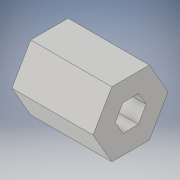
# Autodesk Inventor part: 5mm-.5in hex converter
Saved by Autodesk Inventor 2019 (Build 230136000, 136)
## iProperties
Created: 2020-09-24
Part Number: 5mm-.5in hex converter
Material: Generic
Document SubType Name: Modeling
Designer: User
Density: 1 g/cm^3
Appearance: Default
Author: User
Autodesk Inventor part; units mm, degrees
ref_plane "YZ Plane" through (0, 0, 0) normal (1, 0, 0) x (0, 1, 0)
ref_plane "XZ Plane" through (0, 0, 0) normal (0, 1, 0) x (-1, 0, 0)
ref_plane "XY Plane" through (0, 0, 0) normal (0, 0, 1) x (1, 0, 0)
sketch "Sketch1" plane through (0, 0, 0) normal (1, 0, 0) x (0, 1, 0)
  line L0 (6.35, -3.6662) -> (0, -7.3323)
  line L1 (0, -7.3323) -> (-6.35, -3.6662)
  line L2 (-6.35, -3.6662) -> (-6.35, 3.6662)
  line L3 (-6.35, 3.6662) -> (0, 7.3323)
  line L4 (0, 7.3323) -> (6.35, 3.6662)
  line L5 (6.35, 3.6662) -> (6.35, -3.6662)
  point P0 (0, 0)
  point P1 (0, 0)
  dimension "d0" = 6.35
  constraints: 12 end point, 1 coincident, 13 other
  measures "d0" distance from line of point (0, 0) L5
extrude "Extrusion1" add sketch "Sketch1" along normal blind 3.175
sketch "Sketch3" plane through (0, 0, 0) normal (-1, 0, 0) x (0, 0, 1)
  line L0 (-3.0207, 0.0407) -> (-1.475, 2.6363)
  line L1 (-1.475, 2.6363) -> (1.5456, 2.5956)
  line L2 (1.5456, 2.5956) -> (3.0207, -0.0407)
  line L3 (3.0207, -0.0407) -> (1.475, -2.6363)
  line L4 (1.475, -2.6363) -> (-1.5456, -2.5956)
  line L5 (-1.5456, -2.5956) -> (-3.0207, 0.0407)
  line L6 (-3.6662, 6.35) -> (-7.3323, 0) projected
  line L7 (-7.3323, 0) -> (-3.6662, -6.35) projected
  line L8 (-3.6662, -6.35) -> (3.6662, -6.35) projected
  line L9 (3.6662, -6.35) -> (7.3323, 0) projected
  line L10 (7.3323, 0) -> (3.6662, 6.35) projected
  line L11 (3.6662, 6.35) -> (-3.6662, 6.35) projected
  point P0 (0, 0)
  point P1 (0, 0)
  point P2 (0, 0)
  dimension "d6" = 2.6162
  constraints: 12 end point, 2 coincident, 13 other
  measures "d6" distance from line of L1 point (0, 0)
extrude "Extrusion3" add sketch "Sketch3" along normal blind 12.7
extrude "Extrusion4" cut sketch "Sketch3" against normal through all contours L0 L1 L2 L3 L4 L5
body "Solid1"
